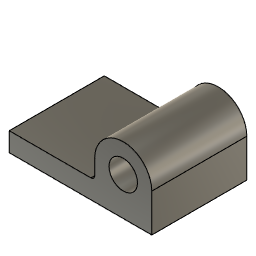
Tutorial Part 4 v3 (Autodesk Fusion 360 design; units mm, degrees)
Autodesk Fusion 360 part; units mm, degrees
sketch "Sketch1" plane through (0, 0, 0) normal (0, 1, 0) x (1, 0, 0)
  line L0 (30, 40) -> (-120, 40)
  line L1 (-120, 40) -> (-120, 20)
  line L2 (-120, 20) -> (-30, 20)
  line L3 (-30, 20) -> (-30, 0)
  arc A0 (-30, 0) -> (30, 0) centre (0, 0) ccw
  line L4 (30, 0) -> (30, 40)
  dimension "d3" = 30
  dimension "d4" = 150
  dimension "d5" = 20
  dimension "d6" = 40
  constraint horizontal L0
  constraint perpendicular L0 L1
  constraint perpendicular L1 L2
  constraint perpendicular L0 L3
  constraint tangent L3 A0
  constraint vertical L4
  constraint tangent A0 L4
  constraint coincident A0.centre origin
  measures "d3" radius of A0
  measures "d4" distance of L0.start L0.end
  measures "d5" distance of L0.end L1.end
  measures "d6" distance of L0 A0.centre
extrude "Extrude1" add sketch "Sketch1" along normal blind 100
fillet "Fillet1" radius 4 1 edges at (-30, 50, -20)
sketch "Sketch2" plane through (0, 0, 0) normal (0, -1, 0) x (1, 0, 0)
  line L0 (30, -40) -> (30, 0)
  arc A0 (30, 0) -> (-30, 0) centre (0, 0) ccw
  line L1 (-30, 0) -> (-30, -16)
  arc A1 (-34, -20) -> (-30, -16) centre (-34, -16) ccw
  line L2 (-34, -20) -> (-120, -20)
  line L3 (-120, -20) -> (-120, -40)
  line L4 (-120, -40) -> (30, -40)
  circle A2 centre (0, 0) radius 15
  dimension "d10" = 30
  constraint coincident A0.centre A2.centre
  measures "d10" diameter of A2
extrude "Extrude2" cut sketch "Sketch2" against normal blind 100 contours A2
